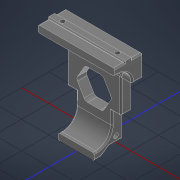
# Autodesk Inventor part: Skirt Front
Saved by Autodesk Inventor 2022.2 (Build 262287010, 287A)
## iProperties
Created: 2022-03-19
Part Number: Skirt Front
Material: ABS-Kunststoff
Document SubType Name: Modeling
Designer: sleib
Density: 1.06 g/cm^3
Appearance: Glatt - Schwarz
Author: sleib
Autodesk Inventor part; units mm, degrees
ref_plane "YZ Plane" through (0, 0, 0) normal (1, 0, 0) x (0, 1, 0)
ref_plane "XZ Plane" through (0, 0, 0) normal (0, 1, 0) x (-1, 0, 0)
ref_plane "XY Plane" through (0, 0, 0) normal (0, 0, 1) x (1, 0, 0)
sketch "Skirt" plane through (0, 0, 0) normal (0, 0, 1) x (1, 0, 0)
  line L0 (33, 20) -> (-33, 20) construction
  line L1 (-33, 20) -> (-33, 0) construction
  line L2 (-33, 0) -> (33, 0) construction
  line L3 (33, 0) -> (33, 20) construction
  line L4 (0, 20) -> (0, 0) construction
  line L5 (33, 20) -> (28, 20)
  line L6 (-33, 20) -> (-28, 20)
  line L7 (33, 20) -> (33, 13)
  line L8 (33, 0) -> (33, 7)
  line L9 (33, 13) -> (34, 13)
  line L10 (33, 7) -> (34, 7)
  line L11 (34, 7) -> (34, 13)
  line L12 (-29, 0) -> (-29, 9)
  line L13 (-29, 9) -> (-33, 14.7126)
  line L14 (-33, 20) -> (-33, 14.7126)
  line L15 (-28, 20) -> (-28, 18)
  line L16 (28, 20) -> (28, 18)
  arc A0 (17, 7) -> (28, 18) centre (17, 18) ccw
  arc A1 (-28, 18) -> (-17, 7) centre (-17, 18) ccw
  line L17 (17, 7) -> (-17, 7)
  line L18 (-29, 0) -> (33, 0)
  line L19 (33, 0.4) -> (32.6, 0)
  line L20 (-29, 0.4) -> (-28.6, 0)
  line L21 (33.2, 13) -> (34, 12.2)
  line L22 (34, 7.8002) -> (33.2, 7)
  point P0 (34, 10)
  point P1 (33, 10)
  dimension "d4" = 66
  dimension "d5" = 20
  dimension "d6" = 5
  dimension "d7" = 5
  dimension "d18" = 1
  dimension "d23" = 9
  dimension "d24" = 4
  dimension "d27" = 35
  dimension "d31" = 2
  dimension "d32" = 2
  dimension "d34" = 6
  dimension "d35" = 13
  dimension "d36" = 0.4
  dimension "d37" = 0.4
  dimension "d38" = 0.4
  dimension "d39" = 0.4
  dimension "d40" = 0.2
  dimension "d41" = 0.8
  dimension "d42" = 0.8002
  measures "d4" distance of L5.start L14.start
  measures "d5" distance of L8.start L5.start
  measures "d6" distance of L5.start L16.start
  measures "d7" distance of L14.start L15.start
  measures "d18" distance of L9.start L11.end
  measures "d23" distance of L12.start L12.end
  measures "d24" distance between parallel lines of L12 L14
  measures "d27" angle of L1 L13
  measures "d31" distance of L15.start L15.end
  measures "d32" distance of L16.start L16.end
  measures "d34" distance between parallel lines of L10 L9
  measures "d35" distance between parallel lines of L17 L0
  measures "d36" distance from line of L18 L19.start
  measures "d37" distance from line of L8 L19.end
  measures "d38" distance from line of L18 L20.start
  measures "d39" distance from line of L12 L20.end
  measures "d40" distance from line of L7 L21.start
  measures "d41" distance from line of L21.end L9
  measures "d42" distance from line of L10 L22.start
sketch "Skizze1" plane through (0, 0, 0) normal (1, 0, 0) x (0, 1, 0)
  circle A0 centre (-25, 4) radius 4 construction
  circle A1 centre (-25, 4) radius 1.7
  line L0 (33, 20) -> (-33, 20) construction
  line L1 (-33, 20) -> (-33, 0) construction
  line L2 (-33, 0) -> (33, 0) construction
  line L3 (33, 0) -> (33, 20) construction
  line L4 (0, 20) -> (0, 0) construction
  line L5 (33, 20) -> (28, 20)
  line L6 (-33, 20) -> (-28, 20)
  line L7 (33, 20) -> (33, 13)
  line L8 (33, 0) -> (33, 7)
  line L9 (33, 13) -> (34, 13)
  line L10 (33, 7) -> (34, 7)
  line L11 (34, 7) -> (34, 13)
  line L12 (-29, 0) -> (-29, 9)
  line L13 (-29, 9) -> (-33, 14.7126)
  line L14 (-33, 20) -> (-33, 14.7126)
  line L15 (-28, 20) -> (-28, 18)
  line L16 (28, 20) -> (28, 18)
  arc A2 (17, 7) -> (28, 18) centre (17, 18) ccw
  arc A3 (-28, 18) -> (-17, 7) centre (-17, 18) ccw
  line L17 (17, 7) -> (-17, 7)
  line L18 (-29, 0) -> (33, 0)
  line L19 (33, 0.4) -> (32.6, 0)
  line L20 (-29, 0.4) -> (-28.6, 0)
  line L21 (33.2, 13) -> (34, 12.2)
  line L22 (34, 7.8002) -> (33.2, 7)
  dimension "d43" = 8
  dimension "d44" = 3.4
  constraints: 2 centre point, 1 coincident, 4 other
  measures "d43" diameter of A0
  measures "d44" diameter of A1
extrude "Extrusion1" add sketch "Skizze1" along normal mid plane 56 contours L7 L9 L21 L11 L22 L10 L8 L19 L18 L20 L12 L13 L14 L6 L15 A3 L17 A2 L16 L5
sketch "Skizze2" plane through (28, 32.6, 0) normal (0, 0, -1) x (-1, 0, 0)
  line L0 (0, -65.6) -> (15, -65.6)
  line L1 (15, -65.6) -> (15, -40.6)
  line L2 (15, -40.6) -> (0, -40.6)
  line L3 (0, -40.6) -> (0, -65.6)
  line L4 (56, -65.6) -> (56, -60.6) projected
  line L5 (56, -65.6) -> (41, -65.6)
  line L6 (41, -65.6) -> (41, -40.6)
  line L7 (41, -40.6) -> (56, -40.6)
  line L8 (56, -40.6) -> (56, -65.6)
  line L9 (0, -61.2) -> (0, 0) projected
  line L10 (56, -65.6) -> (0, -65.6) projected
  line L11 (0, -40.6) -> (8.5, -40.6)
  line L12 (8.5, -40.6) -> (8.5, -15.6)
  line L13 (8.5, -15.6) -> (0, -15.6)
  line L14 (0, -15.6) -> (0, -40.6)
  line L15 (56, -40.6) -> (47.5, -40.6)
  line L16 (47.5, -40.6) -> (47.5, -15.6)
  line L17 (47.5, -15.6) -> (56, -15.6)
  line L18 (56, -15.6) -> (56, -40.6)
  line L19 (56, -15.6) -> (0, -15.6) projected
  line L20 (34.5, -21.3417) -> (41, -32.6)
  line L21 (41, -32.6) -> (34.5, -43.8583)
  line L22 (34.5, -43.8583) -> (21.5, -43.8583)
  line L23 (21.5, -43.8583) -> (15, -32.6)
  line L24 (15, -32.6) -> (21.5, -21.3417)
  line L25 (21.5, -21.3417) -> (34.5, -21.3417)
  point P0 (28, -32.6)
  point P1 (28, -32.6)
  dimension "d48" = 25
  dimension "d53" = 4
  dimension "d54" = 5.7417
  dimension "d55" = 26
  dimension "d56" = 39
  constraints: 44 end point, 8 parallel, 6 collinear, 5 horizontal, 4 perpendicular, 1 coincident, 1 point on line, 13 other
  measures "d48" distance between parallel lines of L0 L2
  measures "d53" distance from line of L1.end L23
  measures "d54" distance between parallel lines of L25 L19
  measures "d55" distance between parallel lines of L6 L1
  measures "d56" distance between parallel lines of L16 L12
extrude "Extrusion2" cut sketch "Skizze2" against normal through all contours L3 L2 L1 L0 | L6 L7 L8 L4 L5 | L9 L13 L12 L2 | L16 L17 L18 L7 | L20 L21 L22 L23 L24 L25
fillet "Rundung1" radius 3 6 edges at (6.5, 11.2583, 3.5) (-6.5, 11.2583, 3.5) (-13, 0, 3.5) (-6.5, -11.2583, 3.5) (6.5, -11.2583, 3.5) (13, 0, 3.5)
sketch "Skizze3" plane through (28, 32.6, 0) normal (0, 0, -1) x (-1, 0, 0)
  line L0 (41, -61.2) -> (41, -40.6) projected
  line L1 (41, -40.6) -> (47.5, -40.6) projected
  line L2 (47.5, -40.6) -> (47.5, -15.6) projected
  line L3 (47.5, -15.6) -> (56, -15.6) projected
  line L4 (56, 0) -> (56, -15.6) projected
  line L5 (56, 0) -> (0, 0) projected
  line L6 (0, -15.6) -> (0, 0) projected
  line L7 (0, -15.6) -> (8.5, -15.6) projected
  line L8 (8.5, -15.6) -> (8.5, -40.6) projected
  line L9 (8.5, -40.6) -> (15, -40.6) projected
  line L10 (15, -40.6) -> (15, -61.2) projected
  line L11 (41, -61.2) -> (15, -61.2) projected
  line L12 (20.634, -42.3583) -> (15.866, -34.1) projected
  arc A0 (15.866, -31.1) -> (15.866, -34.1) centre (18.4641, -32.6) ccw projected
  line L13 (15.866, -31.1) -> (20.634, -22.8417) projected
  arc A1 (23.2321, -21.3417) -> (20.634, -22.8417) centre (23.2321, -24.3417) ccw projected
  line L14 (23.2321, -21.3417) -> (32.7679, -21.3417) projected
  arc A2 (35.366, -22.8417) -> (32.7679, -21.3417) centre (32.7679, -24.3417) ccw projected
  line L15 (35.366, -22.8417) -> (40.134, -31.1) projected
  arc A3 (40.134, -34.1) -> (40.134, -31.1) centre (37.5359, -32.6) ccw projected
  line L16 (40.134, -34.1) -> (35.366, -42.3583) projected
  arc A4 (32.7679, -43.8583) -> (35.366, -42.3583) centre (32.7679, -40.8583) ccw projected
  line L17 (32.7679, -43.8583) -> (23.2321, -43.8583) projected
  arc A5 (20.634, -42.3583) -> (23.2321, -43.8583) centre (23.2321, -40.8583) ccw projected
  line L18 (56, 1.4) -> (0, 1.4) projected
  line L19 (0, 0.6) -> (0, 1.4) projected
  line L20 (56, 0.6) -> (0, 0.6) projected
  line L21 (56, 1.4) -> (56, 0.6) projected
  circle A6 centre (15.5, -3.4) radius 2.25
  circle A7 centre (40.5, -3.4) radius 2.25
  line L22 (56, 0) -> (0, 0) projected
  line L23 (28, 0) -> (28, -61.2) construction
  point P0 (28, -32.6)
  dimension "d58" = 4.5
  dimension "d59" = 25
  dimension "d60" = 4
  constraints: 2 centre point, 2 end point, 2 midpoint, 1 equal radius, 1 horizontal alignment, 1 symmetric about line
  measures "d58" diameter of A6
  measures "d59" distance of A7.centre A6.centre
  measures "d60" distance from line of A6.centre L20
extrude "Extrusion3" cut sketch "Skizze3" against normal blind 6 contours A6 | A7
sketch "Skizze4" plane through (-28, 28, 18) normal (0, -1, 0) x (1, 0, 0)
  line L0 (0, -5.8) -> (56, -5.8) projected
  line L1 (56, -10.1998) -> (56, -5.8) projected
  line L2 (0, -10.1998) -> (56, -10.1998) projected
  line L3 (0, -5.8) -> (0, -10.1998) projected
  circle A0 centre (8, -7.9999) radius 1.7
  circle A1 centre (48, -7.9999) radius 1.7
  circle A2 centre (8, -7.9999) radius 3
  circle A3 centre (48, -7.9999) radius 3
  line L4 (0, -7.9999) -> (56, -7.9999) construction
  line L5 (0, -5.8) -> (56, -5.8) construction
  line L6 (28, -5.8) -> (28, -10.1998) construction
  line L7 (0, -10.1998) -> (56, -10.1998) construction
  point P0 (28, -18)
  dimension "d63" = 3.4
  dimension "d64" = 6
  dimension "d65" = 40
  constraints: 4 centre point, 4 end point, 4 midpoint, 2 coincident, 2 equal radius, 1 point on line, 1 symmetric about line
  measures "d63" diameter of A0
  measures "d64" diameter of A2
  measures "d65" distance of A1.centre A0.centre
extrude "Extrusion4" cut sketch "Skizze4" against normal through all contours A0 | A1
extrude "Extrusion5" cut sketch "Skizze4" along normal blind 11 and the other way blind 2 contours A2 L0 | L0 A2 L2 | L2 A2 | A3 L0 | L0 A3 L2 | L2 A3 | A0 | A1
fillet "Rundung2" radius 1 28 edges at (-28, 28, 19) (-28, 24.7782, 10.2218) (28, 28, 19) (28, 24.7782, 10.2218) (-19.5, 4.5, 7) (19.5, 4.5, 7) (-16.25, -8, 7) (16.25, -8, 7) (-13, -24.7782, 10.2218) (-13, -28, 19) (-13, -12.5, 7) (13, -24.7782, 10.2218) (13, -28, 19) (13, -12.5, 7) (-13, -33, 17.3563) (13, -33, 17.3563) (13, -31, 11.8563) (13, -29, 4.7) (-13, -31, 11.8563) (-13, -29, 4.7) (-19.5, -8, 3.5) (19.5, -8, 3.5) (28, 33, 16.5) (28, 33, 3.7) (-28, 33, 16.5) (-28, 33, 3.7) (-28, 17, 3.5) (28, 17, 3.5)
fillet "Rundung3" radius 1 4 edges at (-28, 32.6, 13) (-28, 32.6, 7) (28, 32.6, 13) (28, 32.6, 7)
